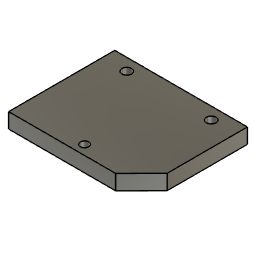
FS40+FS80 Kaiser Klamping Block v3 (Autodesk Fusion 360 design; units mm, degrees)
Autodesk Fusion 360 part; units mm, degrees
sketch "Schizzo1" plane through (0, 0, 0) normal (0, 0, 1) x (1, 0, 0)
  line L0 (24.0483, 47.3102) -> (68.0483, 47.3102)
  line L1 (68.0483, 47.3102) -> (68.0483, 12.1102)
  line L2 (68.0483, 12.1102) -> (24.0483, 12.1102)
  line L3 (24.0483, 12.1102) -> (24.0483, 47.3102)
  line L4 (46.0483, 47.3102) -> (46.0483, 12.1102) construction
  line L5 (24.0483, 43.3102) -> (68.0483, 43.3102) construction
  circle A0 centre (46.0483, 15.3102) radius 1.4
  circle A1 centre (32.0483, 43.3102) radius 1.6
  circle A2 centre (60.0483, 43.3102) radius 1.6
  line L6 (59.5483, 12.1102) -> (68.0483, 20.7102)
  dimension "d1" = 44
  dimension "d2" = 35.2
  dimension "d3" = 2.8
  dimension "d4" = 4
  dimension "d6" = 28
  dimension "d7" = 3.2
  dimension "d8" = 28
  dimension "d9" = 8.5
  dimension "d10" = 8.6
  constraint horizontal L0
  constraint vertical L1
  constraint horizontal L2
  constraint vertical L3
  constraint midpoint L0 L4.start
  constraint midpoint L2 L4.end
  constraint coincident L3 L5.start
  constraint coincident L1 L5.end
  constraint perpendicular L1 L5
  constraint coincident L4 A0.centre
  constraint coincident L5 A1.centre
  constraint symmetric L4 A1 A2
  constraint coincident L2 L6.start
  constraint coincident L1 L6.end
  measures "d1" distance of L0.start L0.end
  measures "d2" distance of L0.start L2.end
  measures "d3" diameter of A0
  measures "d4" distance of L0 L5
  measures "d6" distance of L5 A0.centre
  measures "d7" diameter of A1
  measures "d8" distance of A1.centre A2.centre
  measures "d9" distance of L1.end L6.start
  measures "d10" distance of L1.end L6.end
extrude "Estrusione1" add sketch "Schizzo1" along normal blind 5 contours L0 L1 L2 L3 L6
